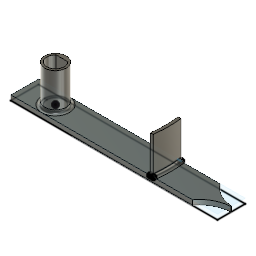
aiguille v5 (Autodesk Fusion 360 design; units mm, degrees)
Autodesk Fusion 360 part; units mm, degrees
sketch "Esquisse1" plane through (0, 0, 0) normal (0, 0, 1) x (1, 0, 0)
  line L0 (-10, 4.5) -> (57, 4.5)
  line L1 (57, 4.5) -> (57, -4.5)
  line L2 (57, -4.5) -> (-10, -4.5)
  line L3 (-10, -4.5) -> (-10, 4.5)
  dimension "d1" = 67
  dimension "d2" = 9
  dimension "d3" = 10
  dimension "d4" = 4.5
  constraint horizontal L0
  constraint vertical L1
  constraint horizontal L2
  constraint vertical L3
  measures "d1" distance of L0.start L0.end
  measures "d2" distance of L0.start L2.end
  measures "d3" horizontal distance of origin L0.start
  measures "d4" vertical distance of origin L0.start
extrude "Extrusion1" add sketch "Esquisse1" along normal blind 1.6
sketch "Esquisse2" plane through (0, 0, 1.6) normal (0, 0, 1) x (-1, 0, 0)
  line L0 (10, 4.5) -> (-57, 4.5)
  line L1 (-57, 4.5) -> (-57, -4.5)
  line L2 (-57, -4.5) -> (10, -4.5)
  line L3 (10, -4.5) -> (10, 4.5)
  circle A0 centre (0, 0) radius 3.5
  arc A1 (-35.2136, 4.5) -> (-35.2135, -4.5007) centre (0, 0) ccw
  arc A2 (-36.2215, 4.5) -> (-36.2215, -4.5) centre (0, 0) ccw
  line L4 (-35.2135, -4.5007) -> (-36.2215, -4.5)
  line L5 (-35.2135, -4.5007) -> (-36.2215, -4.5)
  line L6 (-35.2136, 4.5) -> (-36.2215, 4.5)
  circle A3 centre (0, 0) radius 2.8
  dimension "d7" = 7
  dimension "d8" = 35.5
  dimension "d9" = 36.5
  dimension "d10" = 5.6
  constraint coincident A0.centre A1.centre
  constraint coincident L0 A2.start
  constraint coincident L0 A1.start
  constraint coincident L2 A2.end
  constraint concentric A0 A3
  measures "d7" diameter of A0
  measures "d8" radius of A1
  measures "d9" radius of A2
  measures "d10" diameter of A3
extrude "Extrusion2" add sketch "Esquisse2" along normal blind 12 contours L0 L2 A1 A2 L4 L5 L6
extrude "Extrusion3" add sketch "Esquisse2" along normal blind 12 contours A0
sketch "Esquisse3" plane through (0, 0, 13.6) normal (0, 0, 1) x (-1, 0, 0)
  circle A0 centre (0, 0) radius 2.8
  circle A1 centre (0, 0) radius 3.5
  line L0 (2.0235, -2.7693) -> (-1.9765, -2.7693)
  line L1 (-1.9765, -2.7693) -> (-1.9765, -2.0693)
  line L2 (-1.9765, -2.0693) -> (2.0235, -2.0693)
  line L3 (2.0235, -2.0693) -> (2.0235, -2.7693)
  dimension "d15" = 4
  dimension "d16" = 0.7
  constraint horizontal L0
  constraint vertical L1
  constraint horizontal L2
  constraint vertical L3
  measures "d15" distance of L0.start L0.end
  measures "d16" distance of L0.start L2.end
extrude "Extrusion4" add sketch "Esquisse3" against normal blind 12.2 contours A0 L0 L2 | A0 L0
sketch "Esquisse4" plane through (0, 0, 1.6) normal (0, 0, 1) x (-1, 0, 0)
  circle A0 centre (-57.5342, 10.9) radius 10.7703
  circle A1 centre (-57.5342, -10.9) radius 10.7705
  dimension "d19" = 21.5407
  dimension "d20" = 21.541
  dimension "d21" = 10.9
  dimension "d22" = 10.9
  dimension "d23" = 57.5342
  dimension "d24" = 57.5342
  measures "d19" diameter of A0
  measures "d20" diameter of A1
  measures "d21" vertical distance of A0.centre origin
  measures "d22" vertical distance of A1.centre origin
  measures "d23" horizontal distance of A0.centre origin
  measures "d24" horizontal distance of A1.centre origin
extrude "Extrusion5" cut sketch "Esquisse4" against normal blind 2
fillet "Congé1" radius 1 1 edges at (3.2631, -1.2657, 1.6)
fillet "Congé2" radius 1 2 edges at (35.5, 0, 1.6) (36.5, 0, 1.6)
equation "d23 = 50.53419 mm + 7 mm"
equation "d24 = 50.53419 mm + 7 mm"
